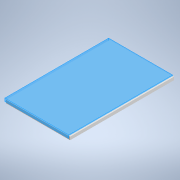
# Autodesk Inventor part: Part1
Saved by Autodesk Inventor 2021 (Build 250183000, 183)
## iProperties
Created: 2020-07-15
Part Number: Part1
Material: Generic
Document SubType Name: Modeling
Designer: adick
Density: 1 g/cm^3
Appearance: Default
Author: adick
Autodesk Inventor part; units mm, degrees
ref_plane "YZ Plane" through (0, 0, 0) normal (1, 0, 0) x (0, 1, 0)
ref_plane "XZ Plane" through (0, 0, 0) normal (0, 1, 0) x (-1, 0, 0)
ref_plane "XY Plane" through (0, 0, 0) normal (0, 0, 1) x (1, 0, 0)
sketch "Sketch1" plane through (0, 0, 0) normal (0, 1, 0) x (-1, 0, 0)
  line L0 (0, 0) -> (265, 0)
  line L1 (265, 0) -> (265, 430)
  line L2 (265, 430) -> (0, 430)
  line L3 (0, 430) -> (0, 0)
  dimension "d1" = 265
  dimension "d2" = 430
  constraints: 8 end point, 2 parallel, 1 horizontal, 1 perpendicular
  measures "d1" distance of L2.end L1.end
  measures "d2" distance of L1.end L0.end
extrude "Extrusion1" add sketch "Sketch1" along normal blind 12.7
body "Solid1"
